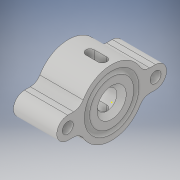
# Autodesk Inventor part: output
Saved by Autodesk Inventor 2018 (Build 220112000, 112)
## iProperties
Created: 2020-03-28
Part Number: output
Material: Generic
Document SubType Name: Modeling
Designer: emile
Density: 1 g/cm^3
Appearance: Default
Author: emile
Autodesk Inventor part; units mm, degrees
ref_plane "YZ Plane" through (0, 0, 0) normal (1, 0, 0) x (0, 1, 0)
ref_plane "XZ Plane" through (0, 0, 0) normal (0, 1, 0) x (-1, 0, 0)
ref_plane "XY Plane" through (0, 0, 0) normal (0, 0, 1) x (1, 0, 0)
sketch "Sketch2" plane through (0, 0, 0) normal (0, 0, 1) x (1, 0, 0)
  line L0 (-28.5524, 19.05) -> (28.5524, 19.05)
  line L1 (28.5524, 19.05) -> (28.5524, 0)
  line L2 (28.5524, 0) -> (-28.5524, 0)
  line L3 (-28.5524, 0) -> (-28.5524, 19.05)
  line L4 (-6.2287, 5.715) -> (-3.4982, 8.4455)
  line L5 (-6.2287, 5.715) -> (-28.5524, 5.715)
  line L6 (-3.4982, 8.4455) -> (0, 8.4455)
  line L7 (0, 8.4455) -> (0, 0)
  line L8 (0, 8.4455) -> (0, 19.05)
  circle A0 centre (0, 0) radius 7.9375 construction
  line L9 (-2.2089, 9.0164) -> (-4.3641, 6.8612) construction
  circle A1 centre (-3.4982, 14.2875) radius 1.524
  line L10 (-7.5974, 2.2987) -> (-28.5524, 2.2987) construction
  line L11 (-25.3774, 5.715) -> (-25.3774, 2.2987)
  line L12 (-25.3774, 0) -> (-25.3774, 2.2987)
  line L13 (-15.8524, 5.715) -> (-15.8524, 2.2987)
  line L14 (-15.8524, 2.54) -> (-25.3774, 2.54)
  line L15 (-3.4982, 8.4455) -> (-3.4982, 19.05)
  dimension "d37" = 15.875
  dimension "d10" = 19.05
  dimension "d35" = 45
  dimension "d36" = 0.508
  dimension "d38" = 5.715
  dimension "d39" = 8.4455
  dimension "d40" = 3.048
  dimension "d41" = 14.2875
  dimension "d43" = 2.2987
  dimension "d44" = 20.955
  dimension "d45" = 3.175
  dimension "d46" = 9.525
  dimension "d47" = 2.54
  constraints: 32 end point, 11 point on line, 7 perpendicular, 3 parallel, 2 coincident, 2 horizontal, 2 midpoint, 1 centre point, 1 collinear, 1 vertical, 1 vertical alignment, 4 other
  measures "d10" distance between parallel lines of L2 L0
  measures "d35" angle of L6 L4
  measures "d36" distance between parallel lines of L4 L9
  measures "d38" distance between parallel lines of L2 L5
  measures "d39" distance between parallel lines of L2 L6
  measures "d40" diameter of A1
  measures "d41" distance from line of L2 A1.centre
  measures "d43" distance between parallel lines of L2 L10
  measures "d44" distance of L10.start L10.end
  measures "d45" distance between parallel lines of L3 L11
  measures "d46" distance between parallel lines of L11 L13
  measures "d47" distance between parallel lines of L2 L14
revolve "Revolution1" add sketch "Sketch2" angle 360 about axis through (28.5524, 0, 0) along (-1, 0, 0) picked at (-3.9732, 14.1074) contours L0 L15 A1 L4 L5 L3 | L5 L11 L12 L2 L3 | L15 A1 | L5 L13 L14 L11
revolve "Revolution2" cut sketch "Sketch2" angle 360 about axis through (28.5524, 0, 0) along (-1, 0, 0) contours L15 A1 | A1 L15
sketch "Sketch5" plane through (-15.8524, 0, 0) normal (1, 0, 0) x (0, 0, -1)
  circle A0 centre (0, 0) radius 5.715 projected
  circle A1 centre (0, 0) radius 2.54 projected
  circle A2 centre (0, 4.064) radius 0.7937
  point P0 (0, 0)
  dimension "d48" = 1.5875
  dimension "d49" = 4.064
  constraints: 1 centre point, 1 vertical alignment
  measures "d48" diameter of A2
  measures "d49" distance of A2.centre point (0, 0)
extrude "Extrusion4" cut sketch "Sketch5" against normal through all contours A2
pattern_circular "Circular Pattern2" count 10 over 360 about axis through (-20.6149, 0, 0) along (1, 0, 0) of "Extrusion4"
sketch "Sketch6" plane through (0, 0, 0) normal (0, 1, 0) x (-1, 0, 0)
  line L0 (6.2287, 5.715) -> (6.2287, -5.715) projected
  line L1 (15.8524, 5.715) -> (15.8524, -5.715) projected
  line L2 (15.8524, 2.54) -> (15.8524, -2.54) projected
  line L3 (25.3774, 2.54) -> (25.3774, -2.54) projected
  line L4 (22.8374, 0) -> (8.7687, 0) construction
  line L5 (22.8374, -2.54) -> (8.7687, -2.54)
  line L6 (8.7687, 2.54) -> (22.8374, 2.54)
  arc A0 (22.8374, -2.54) -> (22.8374, 2.54) centre (22.8374, 0) ccw
  arc A1 (8.7687, 2.54) -> (8.7687, -2.54) centre (8.7687, 0) ccw
  circle A2 centre (15.8031, 0) radius 2.54
  line L7 (15.8031, 0) -> (8.7687, 0) construction
  line L8 (15.8031, 2.54) -> (8.7687, 2.54)
  line L9 (8.7687, -2.54) -> (15.8031, -2.54)
  arc A3 (15.8031, -2.54) -> (15.8031, 2.54) centre (15.8031, 0) ccw
  arc A4 (8.7687, 2.54) -> (8.7687, -2.54) centre (8.7687, 0) ccw
  point P0 (0, 0)
  point P1 (12.2859, 0)
  point P2 (6.2287, 0)
  constraints: 16 end point, 12 tangent, 10 point on circle, 5 centre point, 2 horizontal, 2 horizontal alignment, 2 midpoint, 2 parallel, 1 coincident
extrude "Extrusion5" cut sketch "Sketch6" along normal through all both and the other way through all contours A2 L1 | L1 L5 A2 L6 | A2 L5 A1 L6
sketch "Sketch7" plane through (-15.8524, 0, 0) normal (1, 0, 0) x (0, 0, -1)
  arc A0 (2.5395, 2.5085) -> (2.5395, 4.0671) centre (2.3888, 3.2878) ccw projected
  circle A1 centre (3.8651, 1.2558) radius 0.7937 projected
  circle A2 centre (3.8651, -1.2558) radius 0.7937 projected
  arc A3 (2.5395, -4.0671) -> (2.5395, -2.5085) centre (2.3888, -3.2878) ccw projected
  arc A4 (-2.5395, -2.5085) -> (-2.5395, -4.0671) centre (-2.3888, -3.2878) ccw projected
  circle A5 centre (-3.8651, -1.2558) radius 0.7937 projected
  circle A6 centre (-3.8651, 1.2558) radius 0.7937 projected
  arc A7 (-2.5395, 4.0671) -> (-2.5395, 2.5085) centre (-2.3888, 3.2878) ccw projected
  arc A8 (-2.5395, 5.1198) -> (-2.5395, -5.1198) centre (0, 0) ccw projected
  arc A9 (2.5395, -5.1198) -> (2.5395, 5.1198) centre (0, 0) ccw projected
  spline S0 degree 2 poles (0.7937, 4.064) (0.7937, 5.4388) (-0.3969, 4.7514) (-1.5875, 4.064) (-0.3969, 3.3766) (0.7937, 2.6892) (0.7937, 4.064) knots 0 0 0 0.333333 0.333333 0.666667 0.666667 1 1 1 weights 1 0.5 1 0.5 1 0.5 1 projected
  line L0 (-2.54, -5.1195) -> (-2.54, -18.8799) projected
  line L1 (-2.54, 18.8799) -> (-2.54, 5.1195) projected
  arc A10 (2.5395, 0.0493) -> (-2.5395, 0.0493) centre (0, 0) ccw projected
  line L2 (2.54, -18.8799) -> (2.54, -5.1195) projected
  line L3 (2.54, 5.1195) -> (2.54, 18.8799) projected
  line L4 (2.54, -18.8799) -> (2.54, -5.1195) projected
  line L5 (2.54, 5.1195) -> (2.54, 18.8799) projected
  arc A11 (-2.5395, -0.0493) -> (2.5395, -0.0493) centre (0, 0) ccw projected
  line L6 (-2.54, -5.1195) -> (-2.54, -18.8799) projected
  line L7 (-2.54, 18.8799) -> (-2.54, 5.1195) projected
  spline S1 degree 2 poles (-0.7938, -4.064) (-0.7938, -5.4388) (0.3969, -4.7514) (1.5875, -4.064) (0.3969, -3.3766) (-0.7937, -2.6892) (-0.7938, -4.064) knots 0 0 0 0.333333 0.333333 0.666667 0.666667 1 1 1 weights 1 0.5 1 0.5 1 0.5 1 projected
  arc A12 (0, -5.715) -> (0, 5.715) centre (0, 0) ccw projected
  arc A13 (0, 5.715) -> (0, -5.715) centre (0, 0) ccw projected
  line L8 (-2.5395, 5.1198) -> (-2.54, 5.1195) projected
  line L9 (-2.5395, 4.0671) -> (-2.5395, 5.1198) projected
  line L10 (-2.5395, 0.0493) -> (-2.5395, 2.5085) projected
  arc A14 (2.5395, 0.0493) -> (-2.5395, 0.0493) centre (0, 0) ccw projected
  line L11 (2.5395, 2.5085) -> (2.5395, 0.0493) projected
  line L12 (2.5395, 5.1198) -> (2.5395, 4.0671) projected
  line L13 (2.54, 5.1195) -> (2.5395, 5.1198) projected
  line L14 (2.5395, -5.1198) -> (2.54, -5.1195) projected
  line L15 (2.5395, -4.0671) -> (2.5395, -5.1198) projected
  line L16 (2.5395, -0.0493) -> (2.5395, -2.5085) projected
  line L17 (-2.5395, -2.5085) -> (-2.5395, -0.0493) projected
  line L18 (-2.5395, -5.1198) -> (-2.5395, -4.0671) projected
  line L19 (-2.54, -5.1195) -> (-2.5395, -5.1198) projected
  line L20 (-2.5395, 5.1198) -> (-2.54, 5.1195) projected
  line L21 (-2.5395, 4.0671) -> (-2.5395, 5.1198) projected
  line L22 (-2.5395, 0.0493) -> (-2.5395, 2.5085) projected
  line L23 (2.5395, 2.5085) -> (2.5395, 0.0493) projected
  line L24 (2.5395, 5.1198) -> (2.5395, 4.0671) projected
  line L25 (2.54, 5.1195) -> (2.5395, 5.1198) projected
  line L26 (2.5395, -5.1198) -> (2.54, -5.1195) projected
  line L27 (2.5395, -4.0671) -> (2.5395, -5.1198) projected
  line L28 (2.5395, -0.0493) -> (2.5395, -2.5085) projected
  arc A15 (-2.5395, -0.0493) -> (2.5395, -0.0493) centre (0, 0) ccw projected
  line L29 (-2.5395, -2.5085) -> (-2.5395, -0.0493) projected
  line L30 (-2.5395, -5.1198) -> (-2.5395, -4.0671) projected
  line L31 (-2.54, -5.1195) -> (-2.5395, -5.1198) projected
  line L32 (2.5395, -4.0671) -> (2.5395, -5.1198) projected
  line L33 (2.5395, 5.1198) -> (2.5395, 4.0671) projected
  line L34 (2.5395, 2.5085) -> (2.5395, 0.0493) projected
  arc A16 (2.5395, -0.0493) -> (2.5395, 0.0493) centre (0, 0) ccw projected
  line L35 (2.5395, -0.0493) -> (2.5395, -2.5085) projected
  line L36 (-2.5395, -2.5085) -> (-2.5395, -0.0493) projected
  arc A17 (-2.5395, 0.0493) -> (-2.5395, -0.0493) centre (0, 0) ccw projected
  line L37 (-2.5395, 0.0493) -> (-2.5395, 2.5085) projected
  line L38 (-2.5395, 4.0671) -> (-2.5395, 5.1198) projected
  line L39 (-2.5395, -5.1198) -> (-2.5395, -4.0671) projected
  point P0 (0, 0)
  point P1 (2.54, -5.1195)
  point P2 (2.54, 5.1195)
  point P3 (-2.54, -5.1195)
  point P4 (-2.54, 5.1195)
  constraints: 8 vertical alignment, 4 horizontal alignment, 2 other
extrude "Extrusion6" cut sketch "Sketch7" against normal blind 6.35 contours L11 A10 L10 A7 L9 A13 A12 L12 A0 | A0 L12 A9 L15 A3 L16 A16 L11 | A16 A11 A17 A10 | A17 L17 A4 L18 A8 L9 A7 L10 | L16 A3 L15 A12 A13 L18 A4 L17 A11 | S0 | S1
sketch "Sketch8" plane through (-25.3774, 0, 0) normal (1, 0, 0) x (0, 0, -1)
  circle A0 centre (0, 0) radius 1.905
  point P0 (0, 0)
  dimension "d59" = 3.81
  constraints: 1 centre point, 1 coincident
  measures "d59" diameter of A0
extrude "Extrusion7" cut sketch "Sketch8" against normal through all
sketch "Sketch9" plane through (-3.4982, 0, 0) normal (1, 0, 0) x (0, 0, -1)
  point P0 (0, 0)
sketch "Sketch10" plane through (-3.4982, 0, 0) normal (1, 0, 0) x (0, 0, -1)
  line L0 (-25.4, 6.35) -> (-17.9605, 6.35) projected
  arc A0 (-25.4, 6.35) -> (-25.4, -6.35) centre (-25.4, 0) ccw projected
  line L1 (-25.4, -6.35) -> (-17.9605, -6.35) projected
  circle A1 centre (-25.4, 0) radius 1.5875 projected
  circle A2 centre (0, 0) radius 19.05 projected
  point P0 (0, 0)
extrude "Extrusion8" add sketch "Sketch10" against normal up to surface (25.0541 mm away) contours L0 A2 L1 A0
fillet "Fillet3" radius 6.35 2 edges at (-16.0253, -6.35, 17.9605) (-16.0253, 6.35, 17.9605)
pattern_circular "Circular Pattern3" count 2 over 360 about axis through (-16.0253, 0, 0) along (1, 0, 0) of "Extrusion8", "Fillet3"
sketch "Sketch11" plane through (-3.4982, 0, 25.4) normal (1, 0, 0) x (0, 0, -1)
  circle A0 centre (50.8, 0) radius 1.5875 projected
  circle A1 centre (0, 0) radius 1.5875 projected
  circle A2 centre (25.4, 0) radius 15.8115 projected
  arc A3 (8.9022, -9.525) -> (41.8978, -9.525) centre (25.4, 0) ccw projected
  arc A4 (47.397, -6.35) -> (41.8978, -9.525) centre (47.397, -12.7) ccw projected
  line L0 (47.397, -6.35) -> (50.8, -6.35) projected
  arc A5 (50.8, -6.35) -> (50.8, 6.35) centre (50.8, 0) ccw projected
  line L1 (50.8, 6.35) -> (47.397, 6.35) projected
  arc A6 (41.8978, 9.525) -> (47.397, 6.35) centre (47.397, 12.7) ccw projected
  arc A7 (41.8978, 9.525) -> (8.9022, 9.525) centre (25.4, 0) ccw projected
  arc A8 (3.403, 6.35) -> (8.9022, 9.525) centre (3.403, 12.7) ccw projected
  line L2 (3.403, 6.35) -> (0, 6.35) projected
  arc A9 (0, 6.35) -> (0, -6.35) centre (0, 0) ccw projected
  line L3 (0, -6.35) -> (3.403, -6.35) projected
  arc A10 (8.9022, -9.525) -> (3.403, -6.35) centre (3.403, -12.7) ccw projected
  circle A11 centre (0, 0) radius 3.175
  circle A12 centre (50.8, 0) radius 3.175
  point P0 (25.4, 0)
  dimension "d69" = 6.35
  constraints: 2 centre point, 2 coincident, 1 equal radius
  measures "d69" diameter of A11
extrude "Extrusion9" cut sketch "Sketch11" against normal through all contours A11 | A12
body "Solid2"
